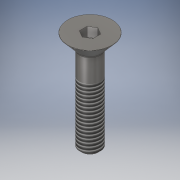
# Autodesk Inventor part: CountersunkBolt
Saved by Autodesk Inventor 2019 (Build 230136000, 136)
## iProperties
Created: 2020-12-09
Part Number: CountersunkBolt
Material: Steel, Carbon
Document SubType Name: Modeling
Designer: Anass Hamdi
Density: 7.85 g/cm^3
Appearance: Semi-Polished
Mass: 3.89322 g
Surface Area: 5.27881 cm^2
Volume: 0.495951 cm^3
Author: Anass Hamdi
Autodesk Inventor part; units mm, degrees
ref_plane "YZ Plane" through (0, 0, 0) normal (1, 0, 0) x (0, 1, 0)
ref_plane "XZ Plane" through (0, 0, 0) normal (0, 1, 0) x (-1, 0, 0)
ref_plane "XY Plane" through (0, 0, 0) normal (0, 0, 1) x (1, 0, 0)
sketch "Sketch1" plane through (0, 0, 0) normal (0, 0, 1) x (1, 0, 0)
  line L0 (0, 0) -> (0, 3.23)
  line L1 (0, 3.23) -> (-5.22, 3.23)
  line L2 (-5.22, 3.23) -> (-5.22, 7.9668) construction
  line L3 (-2.4122, 0) -> (-5.22, 3.23)
  line L4 (0, 0) -> (-2.4122, 0)
  line L5 (-5.22, 3.23) -> (-8.3852, 6.8711) construction
  line L6 (-4.6965, 2.6278) -> (0, 2.6278) construction
  dimension "d0" = 3.23
  dimension "d3" = 41
  dimension "d23" = 5.22
  dimension "d25" = 4.6965
  constraints: 14 end point, 3 perpendicular, 2 point on line, 1 horizontal, 1 vertical
  measures "d0" distance of L0.start L0.end
  measures "d3" angle of L5 L2
  measures "d23" distance of L0.end L1.end
  measures "d25" distance of L6.start L6.end
revolve "Revolution1" add sketch "Sketch1" angle 360 about axis through (0, 0, 0) along (0, 1, 0)
sketch "Sketch2" plane through (0, 0, 0) normal (0, -1, 0) x (1, 0, 0)
  circle A0 centre (0, 0) radius 2.4122 projected
  dimension "d22" = 4.8244
  measures "d22" diameter of A0
extrude "Extrusion1" add sketch "Sketch2" along normal blind 20
sketch "Sketch3" plane through (0, 3.23, 0) normal (0, 1, 0) x (1, 0, 0)
  line L0 (0, -1.836) -> (-1.59, -0.918)
  line L1 (-1.59, -0.918) -> (-1.59, 0.918)
  line L2 (-1.59, 0.918) -> (0, 1.836)
  line L3 (0, 1.836) -> (1.59, 0.918)
  line L4 (1.59, 0.918) -> (1.59, -0.918)
  line L5 (1.59, -0.918) -> (0, -1.836)
  point P0 (0, 0)
  point P1 (0, 0)
  dimension "d8" = 3.18
  constraints: 12 end point, 1 coincident, 13 other
  measures "d8" distance between parallel lines of L1 L4
extrude "Extrusion2" cut sketch "Sketch3" against normal blind 2.21
sketch "Sketch4" plane through (0, 0, 0) normal (0, 0, 1) x (1, 0, 0)
  line L0 (1.59, 1.02) -> (0, 0)
  constraints: 2 end point
sketch "Sketch5" plane through (0, 1.02, 0) normal (0, 1, 0) x (1, 0, 0)
  line L0 (0, -1.836) -> (-1.59, -0.918)
  line L1 (1.59, -0.918) -> (0, -1.836)
  line L2 (1.59, 0.918) -> (1.59, -0.918)
  line L3 (0, 1.836) -> (1.59, 0.918)
  line L4 (-1.59, 0.918) -> (0, 1.836)
  line L5 (-1.59, -0.918) -> (-1.59, 0.918)
  point P0 (0, 0)
  constraints: 12 end point
sketch "Sketch6" plane through (0, 0, 0) normal (0, 1, 0) x (-1, 0, 0)
  point P0 (0, 0)
  point P1 (0, 0)
  constraints: 1 coincident
sketch "Sketch7" plane through (0, 0, 0) normal (1, 0, 0) x (0, 1, 0)
  line L0 (1.02, -1.836) -> (0, 0)
  constraints: 2 end point
loft "Loft1" cut section 1 edges at (-0.795, 1.02, 1.377) (0.795, 1.02, 1.377) (1.59, 1.02, 0) (0.795, 1.02, -1.377) (-0.795, 1.02, -1.377) (-1.59, 1.02, 0) section 2 point at (0, 0, 0)
chamfer "Chamfer1" distance 0.5 angle 45 1 edges at (-2.4122, -20, 0)
thread "Thread1" size "10-32 UNF" class "2A" standard "ANSI Unified Screw Threads" length 14
fillet "Fillet1" radius 0.5 2 edges at (0, 0, -2.4122) (0, 0, 2.4122)
fillet "Fillet2" radius 0.04 1 edges at (5.22, 3.23, 0)
body "Solid1"
